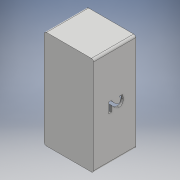
# Autodesk Inventor part: Коробка 2
Saved by Autodesk Inventor 2018 (Build 220112000, 112)
## iProperties
Created: 2023-02-08
Part Number: Коробка 2
Material: Типовые
Document SubType Name: Modeling
Designer: exper
Density: 1 g/cm^3
Appearance: По умолчанию
Author: exper
Autodesk Inventor part; units mm, degrees
ref_plane "YZ Plane" through (0, 0, 0) normal (1, 0, 0) x (0, 1, 0)
ref_plane "XZ Plane" through (0, 0, 0) normal (0, 1, 0) x (-1, 0, 0)
ref_plane "XY Plane" through (0, 0, 0) normal (0, 0, 1) x (1, 0, 0)
sketch "Эскиз1" plane through (0, 0, 0) normal (0, 1, 0) x (-1, 0, 0)
  line L0 (0, 0) -> (-70, 0)
  line L1 (-70, 0) -> (-70, -140)
  line L2 (-70, -140) -> (0, -140)
  line L3 (0, -140) -> (0, 0)
  dimension "d0" = 70
  dimension "d1" = 140
  constraints: 8 end point, 2 parallel, 1 horizontal, 1 perpendicular
  measures "d0" distance of L2.end L1.end
  measures "d1" distance of L1.end L0.end
extrude "Выдавливание1" add sketch "Эскиз1" along normal blind 60
shell "Оболочка1" thickness 3 removed faces 1 at (46.6667, 60, -93.3333)
sketch "Эскиз2" plane through (70, 0, 0) normal (1, 0, 0) x (0, 0, -1)
  line L0 (140, 60) -> (0, 60) projected
  line L1 (60.9522, 42.279) -> (78.4725, 42.279) construction
  line L2 (78.4725, 42.279) -> (78.4725, 21.89) construction
  line L3 (78.4725, 21.89) -> (60.9522, 21.89) construction
  line L4 (60.9522, 21.89) -> (60.9522, 42.279) construction
  line L5 (77.6783, 21.89) -> (62.9781, 21.89)
  line L6 (62.9781, 21.89) -> (62.9781, 25.1477)
  spline S0 degree 2 poles (62.9781, 25.1477) (64.842, 26.6388) (67.8242, 29.2644) (68.9425, 30.4475) knots 0 0 0 1 2 2 2
  spline S1 degree 2 poles (68.9425, 30.4475) (70.4174, 31.9873) (71.7302, 34.3373) (71.7302, 35.5691) knots 0 0 0 1 2 2 2
  spline S2 degree 2 poles (71.7302, 35.5691) (71.7302, 36.9629) (70.0608, 38.454) (68.5697, 38.454) knots 0 0 0 1 2 2 2
  spline S3 degree 2 poles (68.5697, 38.454) (67.808, 38.454) (66.4465, 38.0813) (65.7496, 37.7895) knots 0 0 0 1 2 2 2
  spline S4 degree 2 poles (65.7496, 37.7895) (65.0689, 37.4816) (64.0965, 36.8333) (63.8533, 36.6712) knots 0 0 0 1 2 2 2
  line L7 (63.8533, 36.6712) -> (63.4644, 36.6712)
  line L8 (63.4644, 36.6712) -> (63.4644, 41.031)
  spline S5 degree 2 poles (63.4644, 41.031) (64.3072, 41.4362) (67.9052, 42.279) (69.5746, 42.279) knots 0 0 0 1 2 2 2
  spline S6 degree 2 poles (69.5746, 42.279) (73.1402, 42.279) (76.8031, 39.1023) (76.8031, 36.2336) knots 0 0 0 1 2 2 2
  spline S7 degree 2 poles (76.8031, 36.2336) (76.8031, 34.467) (75.1337, 31.0634) (73.205, 29.1185) knots 0 0 0 1 2 2 2
  spline S8 degree 2 poles (73.205, 29.1185) (71.9895, 27.9192) (69.7042, 26.0553) (69.2018, 25.6663) knots 0 0 0 1 2 2 2
  line L9 (69.2018, 25.6663) -> (77.6783, 25.6663)
  line L10 (77.6783, 25.6663) -> (77.6783, 21.89)
  point P0 (0, 0)
  point P1 (70, 30.6523)
  constraints: 2 other
extrude "Выдавливание2" cut sketch "Эскиз2" against normal blind 30
sketch "Эскиз3" plane through (70, 0, -140) normal (0, 0, -1) x (-1, 0, 0)
  line L0 (67, 60) -> (3, 60) projected
  line L1 (25.4896, 42.8662) -> (43.0099, 42.8662) construction
  line L2 (43.0099, 42.8662) -> (43.0099, 22.4772) construction
  line L3 (43.0099, 22.4772) -> (25.4896, 22.4772) construction
  line L4 (25.4896, 22.4772) -> (25.4896, 42.8662) construction
  line L5 (42.2157, 22.4772) -> (27.5156, 22.4772)
  line L6 (27.5156, 22.4772) -> (27.5156, 25.7349)
  spline S0 degree 2 poles (27.5156, 25.7349) (29.3794, 27.226) (32.3616, 29.8516) (33.4799, 31.0348) knots 0 0 0 1 2 2 2
  spline S1 degree 2 poles (33.4799, 31.0348) (34.9548, 32.5745) (36.2676, 34.9245) (36.2676, 36.1563) knots 0 0 0 1 2 2 2
  spline S2 degree 2 poles (36.2676, 36.1563) (36.2676, 37.5502) (34.5982, 39.0412) (33.1071, 39.0412) knots 0 0 0 1 2 2 2
  spline S3 degree 2 poles (33.1071, 39.0412) (32.3454, 39.0412) (30.9839, 38.6685) (30.287, 38.3767) knots 0 0 0 1 2 2 2
  spline S4 degree 2 poles (30.287, 38.3767) (29.6063, 38.0688) (28.6339, 37.4205) (28.3908, 37.2584) knots 0 0 0 1 2 2 2
  line L7 (28.3908, 37.2584) -> (28.0018, 37.2584)
  line L8 (28.0018, 37.2584) -> (28.0018, 41.6182)
  spline S5 degree 2 poles (28.0018, 41.6182) (28.8446, 42.0234) (32.4426, 42.8662) (34.112, 42.8662) knots 0 0 0 1 2 2 2
  spline S6 degree 2 poles (34.112, 42.8662) (37.6776, 42.8662) (41.3405, 39.6895) (41.3405, 36.8208) knots 0 0 0 1 2 2 2
  spline S7 degree 2 poles (41.3405, 36.8208) (41.3405, 35.0542) (39.6711, 31.6506) (37.7425, 29.7057) knots 0 0 0 1 2 2 2
  spline S8 degree 2 poles (37.7425, 29.7057) (36.5269, 28.5064) (34.2416, 26.6425) (33.7392, 26.2536) knots 0 0 0 1 2 2 2
  line L9 (33.7392, 26.2536) -> (42.2157, 26.2536)
  line L10 (42.2157, 26.2536) -> (42.2157, 22.4772)
  point P0 (70, 0)
  point P1 (35, 32.2964)
  constraints: 2 other
extrude "Выдавливание3" cut sketch "Эскиз3" against normal blind 30
fillet "Сопряжение1" radius 3 4 edges at (3, 31.5, -3) (3, 31.5, -137) (67, 31.5, -3) (67, 31.5, -137)
fillet "Сопряжение2" radius 3 4 edges at (0, 30, -140) (70, 30, -140) (70, 30, 0) (0, 30, 0)
